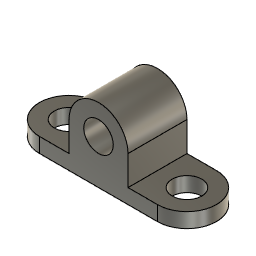
A4 (Autodesk Fusion 360 design; units mm, degrees)
Autodesk Fusion 360 part; units mm, degrees
note: some values were not read from the file. Set by a fixed rule: which sketch regions a step uses.
sketch "Body" plane through (0, 0, 0) normal (0, 0, 1) x (1, 0, 0)
  line L0 (0, 0) -> (80, 0)
  line L1 (80, 0) -> (80, 40)
  line L2 (80, 40) -> (0, 40)
  line L3 (0, 40) -> (0, 0)
  circle A0 centre (0, 20) radius 20
  circle A1 centre (80, 20) radius 20
  line L4 (60, 0) -> (20, 0)
  line L5 (20, 0) -> (20, 40)
  line L6 (20, 40) -> (60, 40)
  line L7 (60, 40) -> (60, 0)
  circle A2 centre (0, 20) radius 10
  circle A3 centre (80, 20) radius 10
  line L8 (40, 40) -> (40, 0) construction
  dimension "d1" = 80
  dimension "d2" = 40
  constraint horizontal L0
  constraint vertical L1
  constraint horizontal L2
  constraint vertical L3
  constraint coincident L0.start L3.end
  constraint midpoint L3 A0.centre
  constraint coincident L0.start A0
  constraint midpoint L1 A1.centre
  constraint coincident L0.end A1
  constraint tangent L0 A1
  constraint horizontal L4
  constraint vertical L5
  constraint horizontal L6
  constraint vertical L7
  constraint coincident L2 L5.end
  constraint coincident L0 L4.start
  constraint concentric A0 A2
  constraint concentric A1 A3
  constraint midpoint L6 L8.start
  constraint midpoint L0 L8.end
  constraint perpendicular L0 L8
  measures "d1" distance of L0.start L0.end
  measures "d2" distance of L0.start L2.end
extrude "Extrude1" add sketch "Body" along normal blind 10
sketch "Circles" plane through (0, 0, 10) normal (0, 0, 1) x (-1, 0, 0)
  arc A0 (0, -40) -> (0, 0) centre (0, -20) ccw
  line L0 (0, 0) -> (-80, 0)
  arc A1 (-80, 0) -> (-80, -40) centre (-80, -20) ccw
  line L1 (-80, -40) -> (0, -40)
  circle A2 centre (-80, -20) radius 20
  circle A3 centre (0, -20) radius 20
  circle A4 centre (0, -20) radius 10
  circle A5 centre (-80, -20) radius 10
  line L2 (-60, 0) -> (-20, 0)
  line L3 (-20, 0) -> (-20, -40)
  line L4 (-20, -40) -> (-60, -40)
  line L5 (-60, -40) -> (-60, 0)
  constraint concentric A3 A4
  constraint concentric A2 A5
  constraint horizontal L2
  constraint vertical L3
  constraint horizontal L4
  constraint vertical L5
  constraint coincident L1 L3.end
  constraint coincident L0 L2.start
extrude "Extrude3" add sketch "Circles" along normal blind 20 contours L0 L1 L2 L3 L4 L5
extrude "Extrude2" cut sketch "Circles" against normal blind 10 contours A4 | A5
sketch "Circles Top" plane through (0, 0, 0) normal (0, -1, 0) x (1, 0, 0)
  line L0 (0, 0) -> (80, 0)
  line L1 (80, 0) -> (80, 10)
  line L2 (80, 10) -> (60, 10)
  line L3 (60, 10) -> (60, 30)
  line L4 (60, 30) -> (20, 30)
  line L5 (20, 30) -> (20, 10)
  line L6 (20, 10) -> (0, 10)
  line L7 (0, 10) -> (0, 0)
  circle A0 centre (40, 30) radius 20
  circle A1 centre (40, 30) radius 10
  constraint midpoint L4 A0.centre
  constraint coincident L3.end A0
  constraint concentric A0 A1
extrude "Extrude5" cut sketch "Circles Top" against normal blind 40 contours L4 A1 picked at (40.2491, 26.676)
extrude "Extrude4" add sketch "Circles Top" against normal blind 40 contours L4 A0 A1 picked at (28.5129, 42.0139)
named bodies: "Object"
